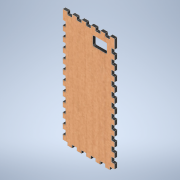
# Autodesk Inventor part: plate_front_big
Saved by Autodesk Inventor 2021 (Build 250183000, 183)
## iProperties
Created: 2021-03-07
Part Number: plate_front_big
Material: Generisch
Document SubType Name: Modeling
Designer: Tilman
Density: 1 g/cm^3
Appearance: Glänzend - Schwarz
Author: Tilman
Autodesk Inventor part; units mm, degrees
ref_plane "YZ Plane" through (0, 0, 0) normal (1, 0, 0) x (0, 1, 0)
ref_plane "XZ Plane" through (0, 0, 0) normal (0, 1, 0) x (-1, 0, 0)
ref_plane "XY Plane" through (0, 0, 0) normal (0, 0, 1) x (1, 0, 0)
sketch "Skizze1" plane through (0, 0, 0) normal (0, 0, 1) x (1, 0, 0)
  line L0 (0, 3) -> (5, 3)
  line L1 (5, 3) -> (5, 0)
  line L2 (5, 0) -> (10, 0)
  line L3 (10, 0) -> (10, 3)
  line L4 (10, 3) -> (15, 3)
  line L5 (15, 3) -> (15, 0)
  line L6 (15, 0) -> (20, 0)
  line L7 (20, 0) -> (20, 3)
  line L8 (20, 3) -> (25, 3)
  line L9 (25, 3) -> (25, 0)
  line L10 (25, 0) -> (30, 0)
  line L11 (30, 0) -> (30, 3)
  line L12 (30, 3) -> (35, 3)
  line L13 (35, 3) -> (35, 0)
  line L14 (35, 0) -> (40, 0)
  line L15 (40, 0) -> (40, 3)
  line L16 (40, 3) -> (45, 3)
  line L17 (45, 3) -> (45, 0)
  line L18 (45, 0) -> (50, 0)
  line L19 (50, 0) -> (50, 3)
  line L20 (50, 3) -> (55, 3)
  line L21 (55, 3) -> (55, 8)
  line L22 (55, 8) -> (52, 8)
  line L23 (52, 8) -> (52, 13)
  line L24 (52, 13) -> (55, 13)
  line L25 (55, 13) -> (55, 18)
  line L26 (52, 18) -> (52, 23)
  line L27 (55, 18) -> (52, 18)
  line L28 (52, 23) -> (55, 23)
  line L29 (55, 23) -> (55, 28)
  line L30 (52, 28) -> (52, 33)
  line L31 (55, 28) -> (52, 28)
  line L32 (52, 33) -> (55, 33)
  line L33 (55, 33) -> (55, 38)
  line L34 (52, 38) -> (52, 43)
  line L35 (55, 38) -> (52, 38)
  line L36 (52, 43) -> (55, 43)
  line L37 (55, 43) -> (55, 48)
  line L38 (52, 48) -> (52, 53)
  line L39 (55, 48) -> (52, 48)
  line L40 (52, 53) -> (55, 53)
  line L41 (55, 53) -> (55, 58)
  line L42 (52, 58) -> (52, 63)
  line L43 (55, 58) -> (52, 58)
  line L44 (52, 63) -> (55, 63)
  line L45 (55, 63) -> (55, 68)
  line L46 (52, 68) -> (52, 73)
  line L47 (55, 68) -> (52, 68)
  line L48 (52, 73) -> (55, 73)
  line L49 (55, 73) -> (55, 78)
  line L50 (52, 78) -> (52, 83)
  line L51 (55, 78) -> (52, 78)
  line L52 (52, 83) -> (55, 83)
  line L53 (55, 83) -> (55, 88)
  line L54 (52, 88) -> (52, 93)
  line L55 (55, 88) -> (52, 88)
  line L56 (52, 93) -> (55, 93)
  line L57 (55, 93) -> (55, 98)
  line L58 (52, 98) -> (52, 103)
  line L59 (55, 98) -> (52, 98)
  line L60 (52, 103) -> (55, 103)
  line L61 (55, 123) -> (50, 123)
  line L62 (50, 123) -> (50, 120)
  line L63 (50, 120) -> (45, 120)
  line L64 (45, 120) -> (45, 123)
  line L65 (40, 120) -> (35, 120)
  line L66 (40, 123) -> (40, 120)
  line L67 (35, 120) -> (35, 123)
  line L68 (45, 123) -> (40, 123)
  line L69 (30, 120) -> (25, 120)
  line L70 (30, 123) -> (30, 120)
  line L71 (25, 120) -> (25, 123)
  line L72 (35, 123) -> (30, 123)
  line L73 (20, 120) -> (15, 120)
  line L74 (20, 123) -> (20, 120)
  line L75 (15, 120) -> (15, 123)
  line L76 (25, 123) -> (20, 123)
  line L77 (10, 120) -> (5, 120)
  line L78 (10, 123) -> (10, 120)
  line L79 (5, 120) -> (5, 123)
  line L80 (15, 123) -> (10, 123)
  line L81 (5, 123) -> (0, 123)
  line L82 (55, 103) -> (55, 108)
  line L83 (52, 108) -> (52, 113)
  line L84 (55, 108) -> (52, 108)
  line L85 (52, 113) -> (55, 113)
  line L86 (55, 123) -> (55, 113)
  line L87 (0, 123) -> (0, 113)
  line L88 (0, 113) -> (3, 113)
  line L89 (3, 113) -> (3, 108)
  line L90 (3, 108) -> (0, 108)
  line L91 (0, 108) -> (0, 103)
  line L92 (3, 103) -> (3, 98)
  line L93 (0, 98) -> (0, 93)
  line L94 (3, 98) -> (0, 98)
  line L95 (0, 103) -> (3, 103)
  line L96 (3, 93) -> (3, 88)
  line L97 (0, 88) -> (0, 83)
  line L98 (3, 88) -> (0, 88)
  line L99 (0, 93) -> (3, 93)
  line L100 (3, 83) -> (3, 78)
  line L101 (0, 78) -> (0, 73)
  line L102 (3, 78) -> (0, 78)
  line L103 (0, 83) -> (3, 83)
  line L104 (3, 73) -> (3, 68)
  line L105 (0, 68) -> (0, 63)
  line L106 (3, 68) -> (0, 68)
  line L107 (0, 73) -> (3, 73)
  line L108 (3, 63) -> (3, 58)
  line L109 (0, 58) -> (0, 53)
  line L110 (3, 58) -> (0, 58)
  line L111 (0, 63) -> (3, 63)
  line L112 (3, 53) -> (3, 48)
  line L113 (0, 48) -> (0, 43)
  line L114 (3, 48) -> (0, 48)
  line L115 (0, 53) -> (3, 53)
  line L116 (3, 43) -> (3, 38)
  line L117 (0, 38) -> (0, 33)
  line L118 (3, 38) -> (0, 38)
  line L119 (0, 43) -> (3, 43)
  line L120 (3, 33) -> (3, 28)
  line L121 (0, 28) -> (0, 23)
  line L122 (3, 28) -> (0, 28)
  line L123 (0, 33) -> (3, 33)
  line L124 (3, 23) -> (3, 18)
  line L125 (0, 18) -> (0, 13)
  line L126 (3, 18) -> (0, 18)
  line L127 (0, 23) -> (3, 23)
  line L128 (3, 13) -> (3, 8)
  line L129 (0, 8) -> (0, 3)
  line L130 (3, 8) -> (0, 8)
  line L131 (0, 13) -> (3, 13)
  line L132 (46, 105) -> (33, 105)
  line L133 (32, 106) -> (32, 114)
  line L134 (33, 115) -> (46, 115)
  line L135 (47, 114) -> (47, 106)
  arc A0 (46, 105) -> (47, 106) centre (46, 106) ccw
  arc A1 (32, 106) -> (33, 105) centre (33, 106) ccw
  arc A2 (33, 115) -> (32, 114) centre (33, 114) ccw
  arc A3 (47, 114) -> (46, 115) centre (46, 114) ccw
  point P0 (0, 0)
  point P1 (47, 105)
  point P2 (32, 115)
  point P3 (32, 105)
  dimension "d0" = 5
  dimension "d1" = 3
  dimension "d4" = 10
  dimension "d11" = 10
  dimension "d18" = 10
  dimension "d32" = 123
  dimension "d35" = 10
  dimension "d40" = 15
  dimension "d41" = 10
  dimension "d42" = 1
  dimension "d43" = 5
  dimension "d44" = 5
  constraints: 272 end point, 29 point on line, 14 equal length, 13 perpendicular, 8 point on circle, 8 tangent, 7 horizontal, 4 centre point, 4 collinear, 4 vertical, 3 equal radius, 3 parallel, 2 vertical alignment, 1 horizontal alignment, 248 other
  measures "d0" distance of L1.end L2.end
  measures "d1" distance of L0.end L1.end
  measures "d4" distance of L0.start L4.start
  measures "d11" distance of L22.end L26.start
  measures "d18" distance of L62.end L65.start
  measures "d32" distance between parallel lines of L14 L72
  measures "d35" distance of L88.end L92.start
  measures "d40" distance of point (47, 105) point (32, 105)
  measures "d41" distance of point (32, 105) point (32, 115)
  measures "d42" radius of A0
  measures "d43" distance between parallel lines of L65 L134
  measures "d44" distance between parallel lines of L83 L135
extrude "Extrusion1" add sketch "Skizze1" along normal blind 3
